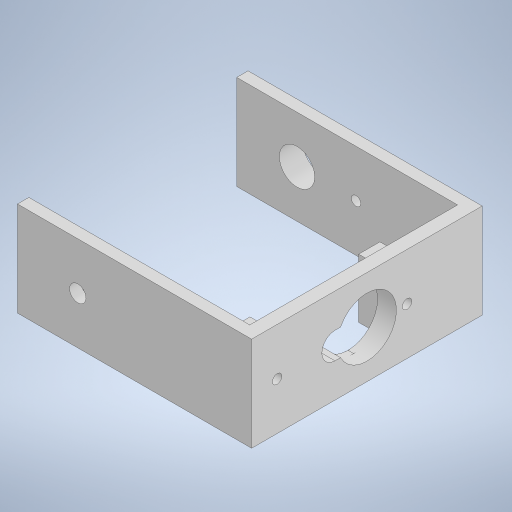
# Autodesk Inventor part: joint3
Saved by Autodesk Inventor 2023 (Build 270158000, 158)
## iProperties
Created: 2023-04-30
Part Number: joint3
Material: 一般
Document SubType Name: Modeling
Designer: taka2
Density: 1 g/cm^3
Appearance: 既定
Author: taka2
Autodesk Inventor part; units mm, degrees
ref_plane "YZ Plane" through (0, 0, 0) normal (1, 0, 0) x (0, 1, 0)
ref_plane "XZ Plane" through (0, 0, 0) normal (0, 1, 0) x (-1, 0, 0)
ref_plane "XY Plane" through (0, 0, 0) normal (0, 0, 1) x (1, 0, 0)
sketch "スケッチ1" plane through (0, 0, 0) normal (0, 1, 0) x (-1, 0, 0)
  line L0 (0, 40.53276) -> (0, -53.904718)
  line L1 (35.916481, 0) -> (-80.691414, 0)
  line L2 (0, -24.4) -> (-49.55, -24.4)
  line L3 (-49.55, -24.4) -> (-49.55, 24.4)
  line L4 (-49.55, 24.4) -> (0, 24.4)
  line L5 (0, 24.4) -> (0, 22)
  line L6 (0, 22) -> (-46.75, 22)
  line L7 (-46.75, 22) -> (-46.75, -22)
  line L8 (-46.75, -22) -> (0, -22)
  line L9 (0, -24.4) -> (0, -22)
  line L10 (-12.75, -24.4) -> (-12.75, 24.4)
  point P0 (0, 0)
  dimension "d0" = 44
  dimension "d1" = 2.4
  dimension "d2" = 12.75
  dimension "d3" = 34
  dimension "d4" = 2.8
  dimension "d5" = 2.4
  constraints: 22 end point, 8 point on line, 4 perpendicular, 3 horizontal, 1 collinear, 1 vertical, 1 other
  measures "d0" distance of L6.end L7.end
  measures "d1" distance of L8.end L2.start
  measures "d2" distance of L10.start L2.start
  measures "d3" horizontal distance of L7.end L10.start
  measures "d4" distance between parallel lines of L3 L7
  measures "d5" distance of L4.end L5.end
sketch "スケッチ1 outline for 押し出し1" plane through (0, 0, 0) normal (0, 1, 0) x (-1, 0, 0)
  line L0 (0, -22) -> (-46.75, -22)
  line L1 (0, -24.4) -> (0, -22)
  line L2 (-49.55, -24.4) -> (0, -24.4)
  line L3 (-49.55, 24.4) -> (-49.55, -24.4)
  line L4 (0, 24.4) -> (-49.55, 24.4)
  line L5 (0, 22) -> (0, 24.4)
  line L6 (-46.75, 22) -> (0, 22)
  line L7 (-46.75, -22) -> (-46.75, 22)
extrude "押し出し1" add sketch "スケッチ1 outline for 押し出し1" along normal blind 20
sketch "スケッチ2" plane through (49.55, 0, -24.4) normal (0, 0, -1) x (-1, 0, 0)
  line L0 (49.55, 20) -> (2.8, 20)
  line L1 (36.8, 20) -> (36.8, 0)
  line L2 (0, 0) -> (49.55, 0)
  line L3 (49.55, 0) -> (49.55, 20)
  line L4 (49.55, 10) -> (0, 10)
  line L5 (0, 0) -> (0, 20)
  circle A0 centre (36.8, 10) radius 3.75
  arc A1 (22.438626, 12.043639) -> (22.438626, 7.956361) centre (22.6, 10) ccw
  line L6 (34.55, 13) -> (22.438626, 12.043639)
  line L7 (34.55, 7) -> (22.438626, 7.956361)
  circle A2 centre (24.3, 10) radius 1
  circle A3 centre (36.8, 10) radius 5.75
  line L8 (33.879857, 14.953309) -> (22.281189, 14.037432)
  arc A4 (22.281189, 14.037432) -> (22.281189, 5.962568) centre (22.6, 10) ccw
  line L9 (22.281189, 5.962568) -> (33.879857, 5.046691)
  dimension "d9" = 7.5
  dimension "d8" = 12.75
  dimension "d10" = 2.05
  dimension "d11" = 14.2
  dimension "d12" = 12.5
  dimension "d13" = 2
  dimension "d14" = 6
  dimension "d43" = 2
  dimension "d44" = 2
  constraints: 12 end point, 6 point on circle, 5 point on line, 4 centre point, 3 midpoint, 2 symmetric about line, 2 tangent, 1 vertical, 4 other
  measures "d8" distance of L0.start L1.start
  measures "d10" radius of A1
  measures "d11" distance of A3.centre A1.centre
  measures "d12" distance of A3.centre A2.centre
  measures "d13" diameter of A2
  measures "d14" distance of L7.start L6.start
  measures "d44" distance between parallel lines of L6 L8
sketch "スケッチ2 outline for 押し出し2" plane through (49.55, 0, -24.4) normal (0, 0, -1) x (-1, 0, 0)
  circle A0 centre (36.8, 10) radius 3.75
  circle A1 centre (24.3, 10) radius 1
extrude "押し出し2" cut sketch "スケッチ2 outline for 押し出し2" against normal up to surface (2.4 mm away)
sketch "スケッチ2 outline for 押し出し7" plane through (49.55, 0, -24.4) normal (0, 0, -1) x (-1, 0, 0)
  arc A0 (33.879857, 5.046691) -> (33.879857, 14.953309) centre (36.8, 10) ccw
  line L0 (22.281189, 5.962568) -> (33.879857, 5.046691)
  line L1 (33.879857, 14.953309) -> (22.281189, 14.037432)
  arc A1 (22.281189, 14.037432) -> (22.281189, 5.962568) centre (22.6, 10) ccw
  arc A2 (34.55, 13) -> (34.55, 7) centre (36.8, 10) cw
  line L2 (22.438626, 12.043639) -> (34.55, 13)
  arc A3 (22.438626, 7.956361) -> (22.438626, 12.043639) centre (22.6, 10) cw
  line L3 (34.55, 7) -> (22.438626, 7.956361)
extrude "押し出し7" add sketch "スケッチ2 outline for 押し出し7" along normal blind 2.6
sketch "スケッチ2 outline for 押し出し3" plane through (49.55, 0, -24.4) normal (0, 0, -1) x (-1, 0, 0)
  arc A0 (34.55, 7) -> (34.55, 13) centre (36.8, 10) cw
  line L0 (22.438626, 7.956361) -> (34.55, 7)
  line L1 (34.55, 13) -> (22.438626, 12.043639)
  arc A1 (22.438626, 12.043639) -> (22.438626, 7.956361) centre (22.6, 10) ccw
  circle A2 centre (24.3, 10) radius 1
extrude "押し出し3" add sketch "スケッチ2 outline for 押し出し3" along normal blind 1.1
sketch "スケッチ3" plane through (0, 0, 24.4) normal (0, 0, 1) x (1, 0, 0)
  circle A0 centre (12.75, 10) radius 3.75 projected
  circle A1 centre (12.75, 10) radius 1.75
  point P0 (0, 0)
  dimension "d19" = 3.5
  constraints: 1 centre point, 1 coincident
  measures "d19" diameter of A1
sketch "スケッチ3 outline for 押し出し4" plane through (0, 0, 24.4) normal (0, 0, 1) x (1, 0, 0)
  circle A0 centre (12.75, 10) radius 1.75
extrude "押し出し4" cut sketch "スケッチ3 outline for 押し出し4" against normal up to surface (2.4 mm away)
sketch "スケッチ4" plane through (46.75, 0, -22) normal (-1, 0, 0) x (0, 0, 1)
  line L0 (22, 0) -> (22, 20)
  line L1 (0, 0) -> (0, 20)
  line L2 (0, 10) -> (44, 10)
  line L3 (44, 0) -> (44, 20)
  line L4 (43.25, 16.25) -> (11.25, 16.25)
  line L5 (11.25, 16.25) -> (11.25, 3.75)
  line L6 (11.25, 3.75) -> (43.25, 3.75)
  line L7 (43.25, 3.75) -> (43.25, 16.25)
  line L8 (15.75, 16.25) -> (15.75, 3.75)
  line L9 (38.75, 16.25) -> (38.75, 3.75)
  circle A0 centre (13.5, 10) radius 1
  circle A1 centre (41, 10) radius 1
  arc A2 (27.58771, 12.8) -> (27.58771, 7.2) centre (22, 10) ccw
  arc A3 (28.75, 7.2) -> (28.75, 12.8) centre (28.75, 10) ccw
  line L10 (28.75, 12.8) -> (27.58771, 12.8)
  line L11 (28.75, 7.2) -> (27.58771, 7.2)
  line L12 (15.75, 3.75) -> (15.75, 10)
  point P0 (22, 10)
  point P1 (15.75, 10)
  point P2 (22, 3.75)
  point P3 (22, 16.25)
  dimension "d22" = 4.5
  dimension "d23" = 4.5
  dimension "d24" = 23
  dimension "d25" = 12.5
  dimension "d29" = 2
  dimension "d30" = 2.25
  dimension "d31" = 2.25
  dimension "d39" = 13
  dimension "d40" = 2.8
  constraints: 22 end point, 7 point on line, 5 point on circle, 4 centre point, 4 midpoint, 4 tangent, 3 horizontal, 3 parallel, 3 perpendicular, 1 equal radius, 1 vertical, 1 other
  measures "d22" distance of L5.end L8.end
  measures "d23" distance of L6.end L9.end
  measures "d24" distance of L9.end L8.end
  measures "d25" distance of L6.end L4.start
  measures "d29" diameter of A1
  measures "d30" distance from line of L7 A1.centre
  measures "d31" distance from line of L5 A0.centre
  measures "d39" distance from line of A3.centre L8
  measures "d40" radius of A3
sketch "スケッチ4 outline for 押し出し5" plane through (46.75, 0, -22) normal (-1, 0, 0) x (0, 0, 1)
  circle A0 centre (41, 10) radius 1
  circle A1 centre (13.5, 10) radius 1
  arc A2 (27.58771, 12.8) -> (27.58771, 7.2) centre (22, 10) ccw
  line L0 (28.75, 12.8) -> (27.58771, 12.8)
  arc A3 (28.75, 7.2) -> (28.75, 12.8) centre (28.75, 10) ccw
  line L1 (27.58771, 7.2) -> (28.75, 7.2)
extrude "押し出し5" cut sketch "スケッチ4 outline for 押し出し5" against normal through all
sketch "スケッチ4 outline for 押し出し8" plane through (46.75, 0, -22) normal (-1, 0, 0) x (0, 0, 1)
  line L0 (15.75, 10) -> (15.75, 3.75)
  arc A0 (22, 3.75) -> (15.75, 10) centre (22, 10) cw
  line L1 (15.75, 3.75) -> (22, 3.75)
  arc A1 (15.75, 10) -> (22, 16.25) centre (22, 10) cw
  line L2 (15.75, 16.25) -> (15.75, 10)
  line L3 (22, 16.25) -> (15.75, 16.25)
  line L4 (28.75, 7.2) -> (27.58771, 7.2)
  arc A2 (28.75, 12.8) -> (28.75, 7.2) centre (28.75, 10) cw
  line L5 (27.58771, 12.8) -> (28.75, 12.8)
  arc A3 (22, 16.25) -> (27.58771, 12.8) centre (22, 10) cw
  line L6 (38.75, 16.25) -> (22, 16.25)
  line L7 (38.75, 3.75) -> (38.75, 16.25)
  line L8 (22, 3.75) -> (38.75, 3.75)
  arc A4 (27.58771, 7.2) -> (22, 3.75) centre (22, 10) cw
extrude "押し出し8" add sketch "スケッチ4 outline for 押し出し8" along normal blind 1.2 contours A0 L1 L0 | L2 L3 A1 | A4 L4 A2 L5 A3 L6 L7 L8
sketch "スケッチ4 outline for 押し出し6" plane through (46.75, 0, -22) normal (-1, 0, 0) x (0, 0, 1)
  line L0 (43.25, 3.75) -> (43.25, 16.25)
  line L1 (38.75, 3.75) -> (43.25, 3.75)
  line L2 (43.25, 16.25) -> (38.75, 16.25)
  line L3 (38.75, 16.25) -> (38.75, 3.75)
  circle A0 centre (41, 10) radius 1
  line L4 (15.75, 3.75) -> (15.75, 16.25)
  line L5 (11.25, 3.75) -> (15.75, 3.75)
  line L6 (15.75, 16.25) -> (11.25, 16.25)
  line L7 (11.25, 16.25) -> (11.25, 3.75)
  circle A1 centre (13.5, 10) radius 1
extrude "押し出し6" add sketch "スケッチ4 outline for 押し出し6" along normal blind 5.2
